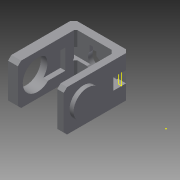
# Autodesk Inventor part: Enlace2
Saved by Autodesk Inventor 2014 SP1 (Build 180222100, 222)
## iProperties
Created: 2013-10-22
Part Number: Enlace2
Material: Genérico
Document SubType Name: Modeling
Designer: Gregorio
Density: 1 g/cm^3
Appearance: Valor por defecto
Author: Gregorio
Autodesk Inventor part; units mm, degrees
ref_plane "YZ Plane" through (0, 0, 0) normal (1, 0, 0) x (0, 1, 0)
ref_plane "XZ Plane" through (0, 0, 0) normal (0, 1, 0) x (-1, 0, 0)
ref_plane "XY Plane" through (0, 0, 0) normal (0, 0, 1) x (1, 0, 0)
sketch "Boceto1" plane through (0, 0, 0) normal (0, 0, 1) x (1, 0, 0)
  line L0 (-27, 0) -> (-31, 0)
  line L1 (-31, 0) -> (-31, 40)
  line L2 (-31, 40) -> (-27, 40)
  line L3 (-27, 40) -> (-27, 0)
  line L4 (-27, 40) -> (-62, 40)
  line L5 (-62, 40) -> (-62, 35.3)
  line L6 (-62, 35.3) -> (-27, 35.3)
  line L7 (-27, 35.3) -> (-27, 40)
  line L8 (-62, 40) -> (-58, 40)
  line L9 (-58, 40) -> (-58, 0)
  line L10 (-58, 0) -> (-62, 0)
  line L11 (-62, 0) -> (-62, 40)
  dimension "d4" = 4
  dimension "d5" = 40
  dimension "d6" = 35
  dimension "d7" = 4.7
  dimension "d8" = 4
  dimension "d9" = 40
  constraints: 24 end point, 6 parallel, 3 horizontal, 3 perpendicular
  measures "d4" distance of L1.end L2.end
  measures "d5" distance of L0.end L1.end
  measures "d6" distance of L6.end L5.end
  measures "d7" distance of L5.end L4.end
  measures "d8" distance of L9.end L10.end
  measures "d9" distance of L8.end L9.end
extrude "Extrusión1" add sketch "Boceto1" along normal blind 25
sketch "Boceto2" plane through (-58, 0, 0) normal (1, 0, 0) x (0, 0, -1)
  line L0 (-25, 0) -> (-25, 35.3) projected
  circle A0 centre (-12.5, 12) radius 9
  line L1 (0, 0) -> (-25, 0) projected
  dimension "d12" = 12.5
  dimension "d13" = 18
  dimension "d21" = 12
  constraints: 1 centre point
  measures "d12" distance from line of L0 A0.centre
  measures "d13" diameter of A0
  measures "d21" distance from line of L1 A0.centre
extrude "Extrusión2" cut sketch "Boceto2" against normal blind 15
sketch "Boceto3" plane through (-27, 0, 0) normal (1, 0, 0) x (0, 0, -1)
  line L0 (0, 0) -> (0, 40) projected
  line L1 (0, 0) -> (-25, 0) projected
  circle A0 centre (-12.5, 12) radius 8.5
  dimension "d16" = 17
  dimension "d17" = 12
  dimension "d18" = 12.5
  constraints: 1 centre point
  measures "d16" diameter of A0
  measures "d17" distance from line of L1 A0.centre
  measures "d18" distance from line of L0 A0.centre
extrude "Extrusión3" add sketch "Boceto3" along normal blind 2.5
sketch "Boceto4" plane through (-58, 0, 0) normal (1, 0, 0) x (0, 0, -1)
  circle A0 centre (-12.5, 12) radius 9 projected
  line L0 (0, 35.3) -> (-25, 35.3) projected
  line L1 (-25, 0) -> (-25, 35.3) projected
  line L2 (0, 0) -> (-25, 0) projected
  line L3 (0, 0) -> (0, 35.3) projected
extrude "Extrusión4" add sketch "Boceto4" along normal blind 4
sketch "Boceto6" plane through (-54, 0, 0) normal (1, 0, 0) x (0, 0, -1)
  line L0 (-18.5, 29) -> (-6.2, 29)
  line L1 (-6.2, 29) -> (-6.2, 5.7)
  line L2 (-6.2, 5.7) -> (-18.5, 5.7)
  line L3 (-18.5, 5.7) -> (-18.5, 29)
  line L4 (-18.5, 29) -> (-18.5, 6) projected
  line L5 (-6.5, 29) -> (-18.5, 29) projected
  dimension "d25" = 12.3
  dimension "d26" = 23.3
  constraints: 8 end point, 2 parallel, 1 collinear, 1 horizontal, 1 perpendicular
  measures "d25" distance of L0.start L0.end
  measures "d26" distance of L2.end L0.start
extrude "Extrusión5" cut sketch "Boceto6" against normal blind 4
sketch "Boceto7" plane through (-58, 40, 0) normal (0, 1, 0) x (1, 0, 0)
  line L0 (31, 0) -> (-4, 0) projected
  circle A0 centre (13.5, -12.5) radius 5
  line L1 (-5, -9) -> (32, -9)
  line L2 (32, -9) -> (32, -16)
  line L3 (32, -16) -> (-5, -16)
  line L4 (-5, -16) -> (-5, -9)
  line L5 (11.5, -4) -> (15.5, -4)
  line L6 (15.5, -4) -> (15.5, -21)
  line L7 (15.5, -21) -> (11.5, -21)
  line L8 (11.5, -21) -> (11.5, -4)
  point P0 (39, 0)
  point P1 (0, 0)
  point P2 (58, 0)
  point P3 (-5, -12.5)
  point P4 (13.5, -9)
  point P5 (11.5, -12.5)
  point P6 (13.5, -4)
  point P7 (13.5, 0)
  dimension "d29" = 10
  dimension "d30" = 37
  dimension "d31" = 7
  dimension "d32" = 12.5
  dimension "d33" = 4
  dimension "d34" = 17
  constraints: 16 end point, 5 midpoint, 4 parallel, 3 vertical alignment, 2 horizontal, 2 horizontal alignment, 2 perpendicular, 1 centre point
  measures "d29" diameter of A0
  measures "d30" distance of L2.end L3.end
  measures "d31" distance of L3.end L1.start
  measures "d32" distance from line of L0 A0.centre
  measures "d33" distance of L6.end L7.end
  measures "d34" distance of L7.end L5.start
extrude "Extrusión6" cut sketch "Boceto7" against normal blind 10 contours A0 L3 L6 L1 | L1 L6 A0 | A0 L6 L3 | L6 L1 L8 A0 | L6 L3 L8 L1 | A0 L8 L3 L6 | L8 L1 A0 | L8 L3 A0 L1 | A0 L3 L8
sketch "Boceto8" plane through (-31, 35.3, 0) normal (0, -1, 0) x (1, 0, 0)
  line L0 (-32, 9) -> (5, 9) projected
  line L1 (-32, 16) -> (-32, 9) projected
  line L2 (5, 16) -> (-32, 16) projected
  line L3 (5, 9) -> (5, 16) projected
  circle A0 centre (-13.5, 12.5) radius 5 projected
  line L4 (-15.5, 21) -> (-15.5, 4) projected
  line L5 (-15.5, 4) -> (-11.5, 4) projected
  line L6 (-11.5, 4) -> (-11.5, 21) projected
  line L7 (-11.5, 21) -> (-15.5, 21) projected
  point P0 (31, 0)
extrude "Extrusión8" cut sketch "Boceto8" against normal blind 2 contours L1 L2 A0 L0 | A0 L2 L4 L0 | L4 L2 L6 L0 | L6 L2 A0 L0 | A0 L2 L3 L0
sketch "Boceto9" plane through (-31, 35.3, 0) normal (0, -1, 0) x (1, 0, 0)
  line L0 (-11.5, 4) -> (-11.5, 21) projected
  line L1 (-15.5, 21) -> (-15.5, 4) projected
  line L2 (-15.5, 4) -> (-11.5, 4) projected
  line L3 (-11.5, 21) -> (-15.5, 21) projected
  point P0 (31, 0)
extrude "Extrusión9" cut sketch "Boceto9" against normal blind 2
sketch "Boceto10" plane through (-54, 0, 0) normal (1, 0, 0) x (0, 0, -1)
  line L0 (-16, 35.3) -> (-9, 35.3)
  line L1 (-9, 35.3) -> (-9, 33.8686)
  line L2 (-9, 33.8686) -> (-16, 33.8686)
  line L3 (-16, 33.8686) -> (-16, 35.3)
  dimension "d43" = 7
  dimension "d44" = 1.4314
  constraints: 8 end point, 2 parallel, 1 horizontal, 1 perpendicular
  measures "d43" distance of L1.end L2.end
  measures "d44" distance of L0.end L1.end
extrude "Extrusión10" cut sketch "Boceto10" against normal blind 2
chamfer "Chaflán3" distance 2 angle 45 3 edges at (-31, 35.3, 4.5) (-31, 35.3, 12.5) (-31, 35.3, 20.5)
chamfer "Chaflán4" distance 2 angle 45 1 edges at (-27, 40, 12.5)
sketch "Boceto11" plane through (-31, 35.3, 0) normal (0, 1, 0) x (1, 0, 0)
  line L0 (2, -16) -> (2, -9) projected
  line L1 (4, -16) -> (2, -16) projected
  line L2 (4, -9) -> (4, -16) projected
  line L3 (2, -9) -> (4, -9) projected
  point P0 (31, 0)
sketch "Boceto12" plane through (-31, 33.3, 9) normal (-0.7071068, 0.7071068, 0) x (-0.7071068, -0.7071068, 0)
  line L0 (0, 0) -> (-2.8284, 0) projected
  line L1 (0, 0) -> (0, 7) projected
  line L2 (0, 7) -> (-2.8284, 7) projected
  line L3 (-2.8284, 7) -> (-2.8284, 0) projected
  point P0 (1.6263, -9)
extrude "Extrusión11" cut sketch "Boceto12" against normal blind 5
sketch "Boceto13" plane through (-27, 0, 25) normal (1, 0, 0) x (0, 0, -1)
  line L0 (9, 30.2289) -> (9, 33.3) projected
  line L1 (9, 33.3) -> (16, 33.3) projected
  line L2 (16, 33.3) -> (16, 30.2289) projected
  line L3 (16, 30.2289) -> (9, 30.2289) projected
  line L4 (9, 30.2289) -> (16, 30.2289)
  line L5 (16, 30.2289) -> (16, 38)
  line L6 (16, 38) -> (9, 38)
  line L7 (9, 38) -> (9, 30.2289)
  dimension "d70" = 7
  constraints: 8 end point, 2 parallel, 1 horizontal, 1 perpendicular
  measures "d70" distance of L2.end L0.start
extrude "Extrusión12" cut sketch "Boceto13" against normal blind 5
sketch "Boceto14" plane through (-62, 0, 0) normal (-1, 0, 0) x (0, 0, 1)
  line L0 (9, 35.3) -> (9, 37.3) projected
  line L1 (9, 37.3) -> (16, 37.3) projected
  line L2 (16, 37.3) -> (16, 35.3) projected
  line L3 (16, 35.3) -> (9, 35.3) projected
  circle A0 centre (12.5, 12) radius 9 projected
  line L4 (25, 40) -> (25, 0) projected
  line L5 (0, 40) -> (25, 40) projected
  line L6 (0, 40) -> (0, 0) projected
  line L7 (0, 0) -> (25, 0) projected
  circle A1 centre (12.5, 12) radius 10
  constraints: 1 centre point, 1 coincident
extrude "Extrusión13" cut sketch "Boceto14" against normal blind 1 contours L4 L7 L6 L5
chamfer "Chaflán8" distance 2 angle 45 1 edges at (-61, 40, 12.5)
sketch "Boceto15" plane through (-54, 0, 0) normal (1, 0, 0) x (0, 0, -1)
  line L0 (-18.5, 18.7082) -> (-18.5, 29) projected
  line L1 (-18.5, 29) -> (-6.2, 29) projected
  line L2 (-6.2, 29) -> (-6.2, 18.4273) projected
  arc A0 (-18.5, 18.7082) -> (-6.2, 18.4273) centre (-12.5, 12) ccw projected
  line L3 (-9, 35.3) -> (-9, 33.8686) projected
  line L4 (-9, 33.8686) -> (-16, 33.8686) projected
  line L5 (-16, 33.8686) -> (-16, 35.3) projected
  line L6 (-25, 35.3) -> (-16, 35.3) projected
  line L7 (-25, 35.3) -> (-25, 0) projected
  line L8 (-25, 0) -> (0, 0) projected
  line L9 (0, 0) -> (0, 35.3) projected
  line L10 (-9, 35.3) -> (0, 35.3) projected
extrude "Extrusión14" cut sketch "Boceto15" against normal blind 1
chamfer "Chaflán9" distance 1 angle 45 2 edges at (-55, 35.3, 4.5) (-55, 35.3, 20.5)
chamfer "Chaflán10" distance 2 angle 45 4 edges at (-29, 0, 25) (-29, 0, 0) (-58, 0, 25) (-58, 0, 0)
